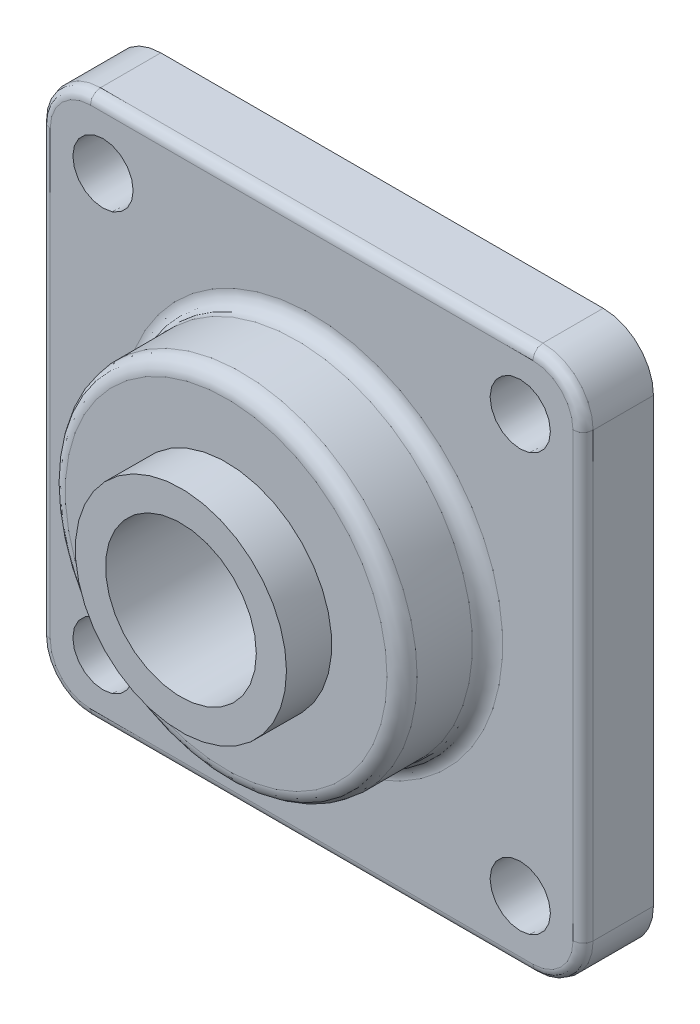
# Autodesk Inventor part: NDM-VOS dummy Disc Harrow Pillow block bearing mount Assembly
Saved by Autodesk Inventor 2025.1 (Build 291241020, 241B)
## iProperties
Created: 2025-01-14
Part Number: NDM-VOS dummy Disc Harrow Pillow block bearing mount Assembly
Material: Generic
Document SubType Name: Modeling
Designer: user
Density: 1 g/cm^3
Appearance: Default
Author: user
Autodesk Inventor part; units mm, degrees
ref_plane "YZ Plane" through (0, 0, 0) normal (1, 0, 0) x (0, 1, 0)
ref_plane "XZ Plane" through (0, 0, 0) normal (0, 1, 0) x (-1, 0, 0)
ref_plane "XY Plane" through (0, 0, 0) normal (0, 0, 1) x (1, 0, 0)
sketch "Sketch1" plane through (0, 0, 0) normal (0, 0, 1) x (1, 0, 0)
  line L0 (-54, 54) -> (54, 54)
  line L1 (54, 54) -> (54, -54)
  line L2 (54, -54) -> (-54, -54)
  line L3 (-54, -54) -> (-54, 54)
  line L4 (-54, 54) -> (54, -54) construction
  line L5 (54, 54) -> (-54, -54) construction
  point P0 (0, 0)
  dimension "d0" = 108
  constraints: 12 end point, 2 midpoint, 2 parallel, 2 perpendicular, 1 horizontal
  measures "d0" distance of L1.end L2.end
extrude "Extrusion1" add sketch "Sketch1" along normal blind 14
sketch "Sketch2" plane through (0, 0, 14) normal (0, 0, 1) x (1, 0, 0)
  circle A0 centre (-41.5, 41.5) radius 6
  line L0 (54, 54) -> (-54, 54) construction
  line L1 (-54, 54) -> (0, 0) construction
  dimension "d4" = 41.5
  dimension "d5" = 12
  constraints: 2 end point, 1 centre point, 1 point on line
  measures "d4" horizontal distance of L1.end A0.centre
  measures "d5" diameter of A0
extrude "Extrusion2" cut sketch "Sketch2" against normal through all
pattern_circular "Circular Pattern1" count 4 over 360 about axis through (0, 0, -10) along (0, 0, 1) of "Extrusion2"
fillet "Fillet1" radius 10 4 edges at (-54, 54, 7) (54, 54, 7) (-54, -54, 7) (54, -54, 7)
sketch "Sketch4" plane through (0, 0, 0) normal (0, 0, 1) x (1, 0, 0)
  circle A0 centre (0, 0) radius 35
  dimension "d15" = 70
  constraints: 1 centre point, 1 coincident
  measures "d15" diameter of A0
extrude "Extrusion4" add sketch "Sketch4" along normal blind 31
sketch "Sketch5" plane through (0, 0, 0) normal (0, 0, 1) x (1, 0, 0)
  circle A0 centre (0, 0) radius 15
  dimension "d18" = 30
  constraints: 1 centre point, 1 coincident
  measures "d18" diameter of A0
extrude "Extrusion5" cut sketch "Sketch5" along normal blind 31
sketch "Sketch6" plane through (0, 0, 0) normal (0, 0, 1) x (1, 0, 0)
  circle A0 centre (0, 0) radius 15 projected
  circle A1 centre (0, 0) radius 21
  dimension "d21" = 6
  constraints: 1 centre point
  measures "d21" radial gap between concentric circles of A0 A1
extrude "Extrusion6" add sketch "Sketch6" along normal blind 40
fillet "Fillet2" radius 3 2 edges at (-35, 0, 31) (-35, 0, 14)
fillet "Fillet3" radius 2 8 edges at (-51.0711, 51.0711, 14) (-54, 0, 14) (-51.0711, -51.0711, 14) (0, -54, 14) (51.0711, -51.0711, 14) (54, 0, 14) (51.0711, 51.0711, 14) (0, 54, 14)
body "Solid1"
